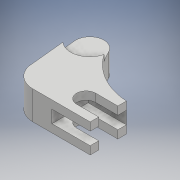
# Autodesk Inventor part: Figure 5.18
Saved by Autodesk Inventor 2018 (Build 220112000, 112)
## iProperties
Created: 2018-01-24
Part Number: Figure 5.18
Material: Generic
Document SubType Name: Modeling
Designer: udyll
Density: 1 g/cm^3
Appearance: Default
Author: udyll
Autodesk Inventor part; units mm, degrees
ref_plane "YZ Plane" through (0, 0, 0) normal (1, 0, 0) x (0, 1, 0)
ref_plane "XZ Plane" through (0, 0, 0) normal (0, 1, 0) x (-1, 0, 0)
ref_plane "XY Plane" through (0, 0, 0) normal (0, 0, 1) x (1, 0, 0)
sketch "Sketch1" plane through (0, 0, 0) normal (0, 0, 1) x (1, 0, 0)
  arc A0 (-22, 0) -> (0, -22) centre (0, 0) ccw
  line L0 (0, 0) -> (49, 0) construction
  arc A1 (0.1199, 52.9967) -> (-26.4108, 44.5873) centre (-12.6821, 47.3304) ccw
  line L1 (-26.6821, 47.3304) -> (-22, 0)
  line L2 (0, -22) -> (57, -22)
  line L3 (57, -22) -> (57, 14)
  arc A2 (0, 53.2602) -> (57, 14) centre (61.0431, 80.8779) ccw
  dimension "d0" = 44
  dimension "d3" = 28
  dimension "d4" = 57
  dimension "d5" = 36
  dimension "d6" = 67
  constraints: 9 point on circle, 8 end point, 3 centre point, 2 horizontal, 1 coincident, 1 perpendicular, 1 point on line, 1 tangent
  measures "d0" diameter of A0
  measures "d3" diameter of A1
  measures "d4" distance of L2.start L2.end
  measures "d5" distance of L2.end L3.end
  measures "d6" radius of A2
extrude "Extrusion1" add sketch "Sketch1" along normal blind 28.52 contours L1 A1 A2 L3 L2 A0
sketch "Sketch2" plane through (0, 0, 28.52) normal (0, 0, 1) x (1, 0, 0)
  arc A0 (0, 53.2602) -> (-26.6821, 47.3304) centre (-12.6821, 47.3304) ccw projected
  circle A1 centre (-12.6821, 47.3304) radius 19
  point P0 (0, 0)
  dimension "d9" = 38
  constraints: 1 centre point, 1 coincident
  measures "d9" diameter of A1
extrude "Extrusion2" cut sketch "Sketch2" against normal blind 6
sketch "Sketch4" plane through (0, 0, 28.52) normal (0, 0, 1) x (1, 0, 0)
  arc A0 (35, 5.525) -> (35, -13.525) centre (35, -4) ccw
  line L0 (35, 5.525) -> (57, 5.525)
  line L1 (35, -13.525) -> (57, -13.525)
  line L2 (57, -22) -> (57, 14) projected
  line L3 (57, 5.525) -> (57, -13.525)
  point P0 (0, 0)
  dimension "d17" = 19.05
  dimension "d19" = 22
  constraints: 6 end point, 2 horizontal, 2 point on circle, 2 point on line, 2 tangent, 1 centre point
  measures "d17" diameter of A0
  measures "d19" distance of L0.start L0.end
extrude "Extrusion3" cut sketch "Sketch4" against normal blind 28.52
sketch "Sketch5" plane through (57, -22, 28.52) normal (1, 0, 0) x (0, 0, -1)
  line L0 (28.52, 36) -> (0, 36) projected
  line L1 (28.52, 36) -> (20.52, 36)
  line L2 (0, 36) -> (8, 36)
  line L3 (0, 0) -> (0, 8.475) projected
  line L4 (0, 0) -> (8, 0)
  line L5 (28.52, 0) -> (0, 0) projected
  line L6 (0, 0) -> (8, 0) construction
  line L7 (28.52, 0) -> (20.52, 0)
  line L8 (8, 36) -> (20.52, 36)
  line L9 (20.52, 36) -> (20.52, 0)
  line L10 (20.52, 0) -> (8, 0)
  line L11 (8, 0) -> (8, 36)
  point P0 (28.52, 22)
  dimension "d22" = 8
  dimension "d23" = 8
  dimension "d24" = 8
  dimension "d25" = 0
  dimension "d26" = 8
  dimension "d27" = 12.52
  constraints: 18 end point, 3 point on line, 2 collinear, 2 horizontal, 2 parallel, 1 perpendicular
  measures "d22" distance of L0.start L1.end
  measures "d23" distance of L0.end L2.end
  measures "d24" distance of L3.start L4.end
  measures "d25" distance between parallel lines of L4 L6
  measures "d26" distance of L5.start L7.end
  measures "d27" distance of L7.end L4.end
extrude "Extrusion4" cut sketch "Sketch5" against normal blind 38
body "Solid1"
